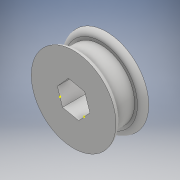
# Autodesk Inventor part: motor gear
Saved by Autodesk Inventor 2018 (Build 220112000, 112)
## iProperties
Created: 2019-11-11
Part Number: motor gear
Material: 일반
Document SubType Name: Modeling
Designer: LeeYounSeo
Density: 1 g/cm^3
Appearance: 기본값
Author: LeeYounSeo
Autodesk Inventor part; units mm, degrees
ref_plane "YZ Plane" through (0, 0, 0) normal (1, 0, 0) x (0, 1, 0)
ref_plane "XZ Plane" through (0, 0, 0) normal (0, 1, 0) x (-1, 0, 0)
ref_plane "XY Plane" through (0, 0, 0) normal (0, 0, 1) x (1, 0, 0)
sketch "스케치1" plane through (0, 0, 0) normal (0, 1, 0) x (-1, 0, 0)
  line L0 (-0.9169, -2.7981) -> (-2.8817, -0.6049)
  line L1 (-2.8817, -0.6049) -> (-1.9647, 2.1931)
  line L2 (-1.9647, 2.1931) -> (0.9169, 2.7981)
  line L3 (0.9169, 2.7981) -> (2.8817, 0.6049)
  line L4 (2.8817, 0.6049) -> (1.9647, -2.1931)
  line L5 (1.9647, -2.1931) -> (-0.9169, -2.7981)
  circle A0 centre (0, 0) radius 7.5
  dimension "d0" = 5.1
  dimension "d1" = 15
  constraints: 12 end point, 2 coincident, 1 centre point, 13 other
  measures "d0" distance between parallel lines of L2 L5
  measures "d1" diameter of A0
extrude "돌출1" add sketch "스케치1" along normal blind 1
sketch "스케치2" plane through (0, 1, 0) normal (0, 1, 0) x (1, 0, 0)
  circle A0 centre (0, 0) radius 6
  line L0 (2.8817, 0.6049) -> (1.9647, -2.1931) projected
  line L1 (1.9647, -2.1931) -> (-0.9169, -2.7981) projected
  line L2 (-0.9169, -2.7981) -> (-2.8817, -0.6049) projected
  line L3 (-2.8817, -0.6049) -> (-1.9647, 2.1931) projected
  line L4 (-1.9647, 2.1931) -> (0.9169, 2.7981) projected
  line L5 (0.9169, 2.7981) -> (2.8817, 0.6049) projected
  circle A1 centre (0, 0) radius 7.5 projected
  dimension "d4" = 12
  constraints: 1 centre point, 1 coincident
  measures "d4" diameter of A0
extrude "돌출2" add sketch "스케치2" along normal blind 3.8 contours A0
sketch "스케치3" plane through (0, 4.8, 0) normal (0, 1, 0) x (1, 0, 0)
  circle A0 centre (0, 0) radius 7.5
  circle A1 centre (0, 0) radius 7.5 projected
  line L0 (1.9647, -2.1931) -> (-0.9169, -2.7981) projected
  line L1 (-0.9169, -2.7981) -> (-2.8817, -0.6049) projected
  line L2 (-2.8817, -0.6049) -> (-1.9647, 2.1931) projected
  line L3 (-1.9647, 2.1931) -> (0.9169, 2.7981) projected
  line L4 (0.9169, 2.7981) -> (2.8817, 0.6049) projected
  line L5 (2.8817, 0.6049) -> (1.9647, -2.1931) projected
  circle A2 centre (0, 0) radius 6 projected
  dimension "d7" = 15
  constraints: 1 centre point, 1 coincident
  measures "d7" diameter of A0
extrude "돌출3" add sketch "스케치3" along normal blind 1 contours A0 | A2
sketch "스케치4" plane through (0, 5.8, 0) normal (0, 1, 0) x (1, 0, 0)
  point P0 (0, 0)
sketch "스케치5" plane through (0, 5.8, 0) normal (0, 1, 0) x (1, 0, 0)
  circle A0 centre (0, 0) radius 5
  circle A1 centre (0, 0) radius 1
  dimension "d10" = 10
  dimension "d11" = 2
  constraints: 2 centre point, 2 coincident
  measures "d10" diameter of A0
  measures "d11" diameter of A1
extrude "돌출4" add sketch "스케치5" against normal blind 0.8
fillet "모깎기1" radius 1 2 edges at (7.5, 1, 0) (-7.5, 4.8, 0)
sketch "스케치6" plane through (0.9169, 0, -2.7981) normal (-0.7448, 0, 0.6673) x (0.6673, 0, 0.7448)
  point P0 (1.4722, 0)
sketch "스케치7" plane through (-2.8817, 0, 0.6049) normal (0.9503, 0, 0.3114) x (0.3114, 0, -0.9503)
  point P0 (1.4722, 0)
